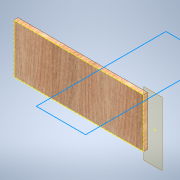
# Autodesk Inventor part: cover
Saved by Autodesk Inventor 2020 (Build 240168000, 168)
## iProperties
Created: 2020-02-17
Part Number: cover
Material: Wood (Birch)
Document SubType Name: Modeling
Designer: erwin
Density: 0.55 g/cm^3
Appearance: Birch - Natural Polished
Author: erwin
Autodesk Inventor part; units mm, degrees
ref_plane "YZ Plane" through (0, 0, 0) normal (1, 0, 0) x (0, 1, 0)
ref_plane "XZ Plane" through (0, 0, 0) normal (0, 1, 0) x (-1, 0, 0)
ref_plane "XY Plane" through (0, 0, 0) normal (0, 0, 1) x (1, 0, 0)
ref_plane "Work Plane1" through (0, 0, 0) normal (0, 0, 1) x (1, 0, 0)
sketch "Sketch1" plane through (0, 0, 0) normal (0, 0, 1) x (1, 0, 0)
  line L0 (-426.9514, -75) -> (-31.8264, 75) construction
  line L1 (-426.9514, 75) -> (-31.8264, -75) construction
  line L2 (-423.9625, 74) -> (-34.8153, 74)
  line L3 (-34.8153, 74) -> (-34.8153, -74)
  line L4 (-34.8153, -74) -> (-423.9625, -74)
  line L5 (-423.9625, -74) -> (-423.9625, 74)
  line L6 (-423.9625, 74) -> (-34.8153, -74) construction
  line L7 (-34.8153, 74) -> (-423.9625, -74) construction
  line L8 (-426.9514, 75) -> (-31.8264, 75) projected
  line L9 (-31.8153, -75) -> (-31.8153, 75) projected
  point P0 (0, 0)
  point P1 (-229.3889, 0)
  dimension "d0" = 1
  dimension "d1" = 3
  constraints: 16 end point, 3 midpoint, 2 parallel, 1 horizontal, 1 perpendicular, 4 other
  measures "d0" distance between parallel lines of L8 L2
  measures "d1" distance between parallel lines of L9 L3
extrude "Extrusion1" add sketch "Sketch1" against normal blind 12
sketch "Sketch2" plane through (0, 0, 0) normal (0, 0, 1) x (1, 0, 0)
  line L0 (-34.8153, -74) -> (-34.8153, 74) projected
  line L1 (-34.8153, 74) -> (-423.9625, 74) projected
  line L2 (-423.9625, 74) -> (-423.9625, -74) projected
  line L3 (-423.9625, -74) -> (-34.8153, -74) projected
  point P0 (0, 0)
body "Solid1"
